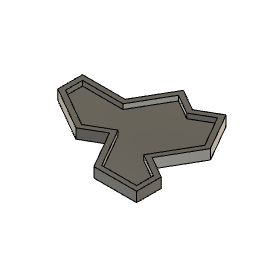
EHK Einstein Tile v2 (Autodesk Fusion 360 design; units mm, degrees)
Autodesk Fusion 360 part; units mm, degrees
sketch "Sketch1" plane through (0, 0, 0) normal (0, 0, 1) x (1, 0, 0)
  line L0 (0, 0) -> (8.6603, 0)
  line L1 (8.6603, 0) -> (8.6603, 5)
  line L2 (8.6603, 5) -> (4.3301, 7.5)
  line L3 (4.3301, 7.5) -> (0, 0)
  line L4 (8.6603, 0) -> (8.6603, 5)
  line L5 (0, 0) -> (8.6603, 0)
  line L6 (4.3301, 7.5) -> (0, 0)
  line L7 (8.6603, 5) -> (4.3301, 7.5)
  line L8 (8.6603, 5) -> (12.9904, 7.5)
  line L9 (8.6603, 0) -> (8.6603, 5)
  line L10 (17.3205, 0) -> (8.6603, 0)
  line L11 (12.9904, 7.5) -> (17.3205, 0)
  line L12 (8.6603, 5) -> (12.9904, 7.5)
  line L13 (8.6603, 0) -> (8.6603, 5)
  line L14 (12.9904, 7.5) -> (17.3205, 0)
  line L15 (17.3205, 0) -> (8.6603, 0)
  line L16 (8.6603, -5) -> (4.3301, -7.5)
  line L17 (12.9904, -7.5) -> (17.3205, 0)
  line L18 (8.6603, 0) -> (8.6603, -5)
  line L19 (17.3205, 0) -> (8.6603, 0)
  line L20 (0, 0) -> (8.6603, 0)
  line L21 (0, 0) -> (8.6603, 0)
  line L22 (8.6603, 0) -> (8.6603, -5)
  line L23 (4.3301, -7.5) -> (0, 0)
  line L24 (8.6603, -5) -> (12.9904, -7.5)
  line L25 (17.3205, 0) -> (8.6603, 0)
  line L26 (12.9904, -7.5) -> (17.3205, 0)
  line L27 (8.6603, -5) -> (4.3301, -7.5)
  line L28 (4.3301, -7.5) -> (0, 0)
  line L29 (8.6603, -5) -> (12.9904, -7.5)
  line L30 (8.6603, 0) -> (8.6603, -5)
  line L31 (8.6603, 0) -> (8.6603, -5)
  line L32 (4.3301, -7.5) -> (0, 0)
  line L33 (-4.3301, -7.5) -> (0, -10)
  line L34 (-4.3301, -7.5) -> (-8.6603, -5)
  line L35 (0, -10) -> (4.3301, -7.5)
  line L36 (0, -10) -> (4.3301, -7.5)
  line L37 (-4.3301, -7.5) -> (-8.6603, -5)
  line L38 (4.3301, -7.5) -> (0, 0)
  line L39 (-4.3301, -7.5) -> (-8.6603, -5)
  line L40 (-8.6603, 0) -> (0, 0)
  line L41 (0, 0) -> (-4.3301, -7.5)
  line L42 (-8.6603, -5) -> (-8.6603, 0)
  line L43 (-8.6603, -5) -> (-8.6603, 0)
  line L44 (-4.3301, -7.5) -> (0, -10)
  line L45 (-4.3301, -7.5) -> (0, -10)
  line L46 (0, 0) -> (-4.3301, -7.5)
  line L47 (-4.3301, -7.5) -> (-8.6603, -5)
  line L48 (-8.6603, 0) -> (0, 0)
  line L49 (0, 0) -> (-4.3301, -7.5)
  line L50 (0, 0) -> (-4.3301, -7.5)
  line L51 (-4.3301, -7.5) -> (0, -10)
  line L52 (8.6603, -15) -> (12.9904, -7.5)
  line L53 (8.6603, -15) -> (12.9904, -7.5)
  line L54 (17.3205, -10) -> (17.3205, -15)
  line L55 (8.6603, -15) -> (12.9904, -7.5)
  line L56 (8.6603, -15) -> (12.9904, -7.5)
  line L57 (12.9904, -7.5) -> (8.6603, -5)
  line L58 (12.9904, -7.5) -> (8.6603, -5)
  line L59 (12.9904, -7.5) -> (8.6603, -5)
  line L60 (12.9904, -7.5) -> (8.6603, -5)
  line L61 (12.9904, -7.5) -> (17.3205, -10)
  line L62 (17.3205, -10) -> (17.3205, -15)
  line L63 (12.9904, -7.5) -> (17.3205, -10)
  line L64 (4.3301, -7.5) -> (8.6603, -15)
  line L65 (4.3301, -7.5) -> (8.6603, -15)
  line L66 (12.9904, -7.5) -> (17.3205, -10)
  line L67 (17.3205, -15) -> (8.6603, -15)
  line L68 (12.9904, -7.5) -> (17.3205, -10)
  line L69 (8.6603, -5) -> (4.3301, -7.5)
  line L70 (4.3301, -7.5) -> (8.6603, -15)
  line L71 (17.3205, -15) -> (8.6603, -15)
  line L72 (8.6603, -5) -> (4.3301, -7.5)
  line L73 (4.3301, -7.5) -> (8.6603, -15)
  point P0 (17.3205, 0)
  point P1 (17.3205, 0)
  point P2 (17.3205, 0)
  point P3 (17.3205, 0)
  point P4 (8.6603, -15)
  point P5 (8.6603, -15)
  point P6 (8.6603, -15)
  point P7 (8.6603, -15)
  point P8 (8.6603, -15)
  point P9 (8.6603, -15)
  point P10 (8.6603, -15)
  point P11 (8.6603, -15)
  point P12 (8.6603, -15)
  point P13 (8.6603, -15)
  point P14 (8.6603, -15)
  point P15 (8.6603, -15)
  point P16 (8.6603, -15)
  point P17 (8.6603, -15)
  dimension "d1" = 5
  dimension "d3" = 60
  dimension "d5" = 5
  dimension "d6" = 60
  constraint coincident L0.start L3.end
  constraint horizontal L0
  constraint perpendicular L0 L1
  constraint equal L0 L3
  constraint equal L1 L2
  constraint horizontal L5
  constraint perpendicular L4 L5
  constraint equal L5 L6
  constraint equal L4 L7
  constraint symmetric L0.start L1 P3
  constraint symmetric L0.end L1 L4.start
  constraint symmetric L2.start L1 L4.end
  constraint symmetric L1 L2.end L8.end
  constraint symmetric L1 L0.start P3
  constraint symmetric L1 L0.end L4.start
  constraint symmetric L1 L2.start L4.end
  constraint symmetric L0.start L15 L3.end
  constraint symmetric L0.end L15 L1.start
  constraint symmetric L1.end L15 L16.start
  constraint symmetric L2.end L15 L16.end
  constraint symmetric P3 L15 P2
  constraint symmetric L8.end L15 L17.start
  constraint symmetric L0.start L23 L3.end
  constraint symmetric L0.end L23 L33.start
  constraint symmetric L1.end L23 L34.end
  constraint symmetric L2.end L23 L40.start
  constraint symmetric L16.start L23 L33.end
  constraint symmetric L16.end L23 L27.end
  constraint symmetric L0.start L16 P17
  constraint symmetric L0.end L16 L17.start
  constraint symmetric L1.end L16 L54.start
  constraint symmetric L2.end L16 L54.end
  constraint symmetric L18.end L16 L22.end
  constraint symmetric L23.start L16 L27.end
  constraint symmetric L16 L0.start P17
  constraint symmetric L16 L23.start L27.end
  measures "d1" distance of L0.end L1.end
  measures "d3" angle of L0 L3
  measures "d5" distance of L0.end L1.end
  measures "d6" angle of L5 L6
extrude "Extrude1" add sketch "Sketch1" along normal blind 2
sketch "Sketch2" plane through (0, 0, 2) normal (0, 0, 1) x (-1, 0, 0)
  line L0 (8.6603, 5) -> (0, 10)
  line L1 (0, 10) -> (-4.3301, 7.5)
  line L2 (-4.3301, 7.5) -> (-8.6603, 15)
  line L3 (-8.6603, 15) -> (-17.3205, 15)
  line L4 (-17.3205, 15) -> (-17.3205, 10)
  line L5 (-17.3205, 10) -> (-12.9904, 7.5)
  line L6 (-12.9904, 7.5) -> (-17.3205, 0)
  line L7 (-17.3205, 0) -> (-12.9904, -7.5)
  line L8 (-12.9904, -7.5) -> (-8.6603, -5)
  line L9 (-8.6603, -5) -> (-4.3301, -7.5)
  line L10 (-4.3301, -7.5) -> (0, 0)
  line L11 (0, 0) -> (8.6603, 0)
  line L12 (8.6603, 0) -> (8.6603, 5)
  line L13 (-0.5774, 1) -> (7.6603, 1)
  line L14 (7.6603, 1) -> (7.6603, 4.4226)
  line L15 (7.6603, 4.4226) -> (0, 8.8453)
  line L16 (0, 8.8453) -> (-4.6962, 6.134)
  line L17 (-4.6962, 6.134) -> (-9.2376, 14)
  line L18 (-9.2376, 14) -> (-16.3205, 14)
  line L19 (-16.3205, 14) -> (-16.3205, 10.5774)
  line L20 (-16.3205, 10.5774) -> (-11.6244, 7.866)
  line L21 (-11.6244, 7.866) -> (-16.1658, 0)
  line L22 (-16.1658, 0) -> (-12.6244, -6.134)
  line L23 (-12.6244, -6.134) -> (-8.6603, -3.8453)
  line L24 (-8.6603, -3.8453) -> (-4.6962, -6.134)
  line L25 (-4.6962, -6.134) -> (-0.5774, 1)
  dimension "d9" = -1
extrude "Extrude2" cut sketch "Sketch2" against normal blind 1 contours L13 L14 L15 L16 L17 L18 L19 L20 L21 L22 L23 L24 L25
